Autodesk Inventor part; units mm, degrees
(part 5 of 7)
  arc A1272 (-12.9119, 20.5084) -> (-12.9119, 24.5084) centre (-12.9119, 22.5084) ccw
  arc A1273 (-46.3463, 24.5084) -> (-46.3463, 20.5084) centre (-46.3463, 22.5084) ccw
  arc A1274 (-52.9119, 20.5084) -> (-52.9119, 24.5084) centre (-52.9119, 22.5084) ccw
  arc A1275 (-46.3463, 24.5084) -> (-46.3463, 20.5084) centre (-46.3463, 22.5084) ccw
  arc A1276 (-46.3463, 24.5084) -> (-46.3463, 20.5084) centre (-46.3463, 22.5084) ccw
  arc A1277 (-46.3463, 24.5084) -> (-46.3463, 20.5084) centre (-46.3463, 22.5084) ccw
  arc A1278 (-46.3463, 24.5084) -> (-46.3463, 20.5084) centre (-46.3463, 22.5084) ccw
  arc A1279 (-46.3463, 24.5084) -> (-46.3463, 20.5084) centre (-46.3463, 22.5084) ccw
  arc A1280 (-52.9119, 20.5084) -> (-52.9119, 24.5084) centre (-52.9119, 22.5084) ccw
  arc A1281 (-52.9119, 20.5084) -> (-52.9119, 24.5084) centre (-52.9119, 22.5084) ccw
  arc A1282 (-52.9119, 20.5084) -> (-52.9119, 24.5084) centre (-52.9119, 22.5084) ccw
  arc A1283 (-52.9119, 20.5084) -> (-52.9119, 24.5084) centre (-52.9119, 22.5084) ccw
  line L1132 (-42.4124, 31.4654) -> (-55.8468, 31.4654)
  line L1133 (-55.8468, 27.4654) -> (-42.4124, 27.4654)
  line L1134 (-55.8468, 27.4654) -> (-42.4124, 27.4654)
  line L1135 (-55.8468, 27.4654) -> (-42.4124, 27.4654)
  line L1136 (-55.8468, 27.4654) -> (-42.4124, 27.4654)
  line L1137 (-55.8468, 27.4654) -> (-42.4124, 27.4654)
  line L1138 (-42.4124, 31.4654) -> (-55.8468, 31.4654)
  line L1139 (-42.4124, 31.4654) -> (-55.8468, 31.4654)
  line L1140 (-42.4124, 31.4654) -> (-55.8468, 31.4654)
  line L1141 (-42.4124, 31.4654) -> (-55.8468, 31.4654)
  arc A1284 (-86.3463, 24.5084) -> (-86.3463, 20.5084) centre (-86.3463, 22.5084) ccw
  arc A1285 (-86.3463, 24.5084) -> (-86.3463, 20.5084) centre (-86.3463, 22.5084) ccw
  arc A1286 (-86.3463, 24.5084) -> (-86.3463, 20.5084) centre (-86.3463, 22.5084) ccw
  arc A1287 (-92.9119, 20.5084) -> (-92.9119, 24.5084) centre (-92.9119, 22.5084) ccw
  line L1142 (-82.4124, 31.4654) -> (-95.8468, 31.4654)
  line L1143 (-95.8468, 27.4654) -> (-82.4124, 27.4654)
  line L1144 (-86.3463, 20.5084) -> (-72.9119, 20.5084)
  line L1145 (-86.3463, 20.5084) -> (-72.9119, 20.5084)
  line L1146 (-86.3463, 20.5084) -> (-72.9119, 20.5084)
  line L1147 (-72.9119, 24.5084) -> (-86.3463, 24.5084)
  line L1148 (-72.9119, 24.5084) -> (-86.3463, 24.5084)
  line L1149 (-72.9119, 24.5084) -> (-86.3463, 24.5084)
  arc A1288 (-75.8468, 31.4654) -> (-75.8468, 27.4654) centre (-75.8468, 29.4654) ccw
  arc A1289 (-75.8468, 31.4654) -> (-75.8468, 27.4654) centre (-75.8468, 29.4654) ccw
  arc A1290 (-75.8468, 31.4654) -> (-75.8468, 27.4654) centre (-75.8468, 29.4654) ccw
  arc A1291 (-75.8468, 31.4654) -> (-75.8468, 27.4654) centre (-75.8468, 29.4654) ccw
  arc A1292 (-82.4124, 27.4654) -> (-82.4124, 31.4654) centre (-82.4124, 29.4654) ccw
  line L1150 (-66.3463, 20.5084) -> (-52.9119, 20.5084)
  line L1151 (-52.9119, 24.5084) -> (-66.3463, 24.5084)
  line L1152 (-52.9119, 24.5084) -> (-66.3463, 24.5084)
  line L1153 (-66.3463, 20.5084) -> (-52.9119, 20.5084)
  line L1154 (-52.9119, 24.5084) -> (-66.3463, 24.5084)
  line L1155 (-52.9119, 24.5084) -> (-66.3463, 24.5084)
  line L1156 (-52.9119, 24.5084) -> (-66.3463, 24.5084)
  line L1157 (-66.3463, 20.5084) -> (-52.9119, 20.5084)
  line L1158 (-66.3463, 20.5084) -> (-52.9119, 20.5084)
  line L1159 (-66.3463, 20.5084) -> (-52.9119, 20.5084)
  line L1160 (-46.3463, 20.5084) -> (-32.9119, 20.5084)
  line L1161 (-32.9119, 24.5084) -> (-46.3463, 24.5084)
  line L1162 (-32.9119, 24.5084) -> (-46.3463, 24.5084)
  line L1163 (-46.3463, 20.5084) -> (-32.9119, 20.5084)
  line L1164 (-32.9119, 24.5084) -> (-46.3463, 24.5084)
  line L1165 (-32.9119, 24.5084) -> (-46.3463, 24.5084)
  line L1166 (-32.9119, 24.5084) -> (-46.3463, 24.5084)
  line L1167 (-46.3463, 20.5084) -> (-32.9119, 20.5084)
  line L1168 (-46.3463, 20.5084) -> (-32.9119, 20.5084)
  line L1169 (-46.3463, 20.5084) -> (-32.9119, 20.5084)
  line L1170 (-46.3463, 20.5084) -> (-32.9119, 20.5084)
  line L1171 (-32.9119, 24.5084) -> (-46.3463, 24.5084)
  arc A1293 (-55.8468, 31.4654) -> (-55.8468, 27.4654) centre (-55.8468, 29.4654) ccw
  arc A1294 (-55.8468, 31.4654) -> (-55.8468, 27.4654) centre (-55.8468, 29.4654) ccw
  arc A1295 (-55.8468, 31.4654) -> (-55.8468, 27.4654) centre (-55.8468, 29.4654) ccw
  arc A1296 (-62.4124, 27.4654) -> (-62.4124, 31.4654) centre (-62.4124, 29.4654) ccw
  arc A1297 (-55.8468, 31.4654) -> (-55.8468, 27.4654) centre (-55.8468, 29.4654) ccw
  arc A1298 (-55.8468, 31.4654) -> (-55.8468, 27.4654) centre (-55.8468, 29.4654) ccw
  arc A1299 (-55.8468, 31.4654) -> (-55.8468, 27.4654) centre (-55.8468, 29.4654) ccw
  arc A1300 (-55.8468, 31.4654) -> (-55.8468, 27.4654) centre (-55.8468, 29.4654) ccw
  arc A1301 (-62.4124, 27.4654) -> (-62.4124, 31.4654) centre (-62.4124, 29.4654) ccw
  arc A1302 (-62.4124, 27.4654) -> (-62.4124, 31.4654) centre (-62.4124, 29.4654) ccw
  arc A1303 (-66.3463, 24.5084) -> (-66.3463, 20.5084) centre (-66.3463, 22.5084) ccw
  arc A1304 (-72.9119, 20.5084) -> (-72.9119, 24.5084) centre (-72.9119, 22.5084) ccw
  arc A1305 (-66.3463, 24.5084) -> (-66.3463, 20.5084) centre (-66.3463, 22.5084) ccw
  line L1172 (-62.4124, 31.4654) -> (-75.8468, 31.4654)
  line L1173 (-75.8468, 27.4654) -> (-62.4124, 27.4654)
  arc A1306 (-72.9119, 20.5084) -> (-72.9119, 24.5084) centre (-72.9119, 22.5084) ccw
  line L1174 (-62.4124, 31.4654) -> (-75.8468, 31.4654)
  line L1175 (-75.8468, 27.4654) -> (-62.4124, 27.4654)
  arc A1307 (-66.3463, 24.5084) -> (-66.3463, 20.5084) centre (-66.3463, 22.5084) ccw
  arc A1308 (-66.3463, 24.5084) -> (-66.3463, 20.5084) centre (-66.3463, 22.5084) ccw
  arc A1309 (-66.3463, 24.5084) -> (-66.3463, 20.5084) centre (-66.3463, 22.5084) ccw
  line L1176 (-62.4124, 31.4654) -> (-75.8468, 31.4654)
  line L1177 (-75.8468, 27.4654) -> (-62.4124, 27.4654)
  arc A1310 (-72.9119, 20.5084) -> (-72.9119, 24.5084) centre (-72.9119, 22.5084) ccw
  arc A1311 (-106.3463, 24.5084) -> (-106.3463, 20.5084) centre (-106.3463, 22.5084) ccw
  arc A1312 (-95.8468, 31.4654) -> (-95.8468, 27.4654) centre (-95.8468, 29.4654) ccw
  line L1178 (-92.9119, 24.5084) -> (-106.3463, 24.5084)
  line L1179 (-106.3463, 20.5084) -> (-92.9119, 20.5084)
  arc A1313 (-35.8468, 31.4654) -> (-35.8468, 27.4654) centre (-35.8468, 29.4654) ccw
  arc A1314 (-35.8468, 31.4654) -> (-35.8468, 27.4654) centre (-35.8468, 29.4654) ccw
  arc A1315 (-35.8468, 31.4654) -> (-35.8468, 27.4654) centre (-35.8468, 29.4654) ccw
  arc A1316 (-42.4124, 27.4654) -> (-42.4124, 31.4654) centre (-42.4124, 29.4654) ccw
  arc A1317 (-42.4124, 27.4654) -> (-42.4124, 31.4654) centre (-42.4124, 29.4654) ccw
  arc A1318 (-35.8468, 31.4654) -> (-35.8468, 27.4654) centre (-35.8468, 29.4654) ccw
  arc A1319 (-35.8468, 31.4654) -> (-35.8468, 27.4654) centre (-35.8468, 29.4654) ccw
  arc A1320 (-35.8468, 31.4654) -> (-35.8468, 27.4654) centre (-35.8468, 29.4654) ccw
  arc A1321 (-35.8468, 31.4654) -> (-35.8468, 27.4654) centre (-35.8468, 29.4654) ccw
  arc A1322 (-35.8468, 31.4654) -> (-35.8468, 27.4654) centre (-35.8468, 29.4654) ccw
  arc A1323 (-35.8468, 31.4654) -> (-35.8468, 27.4654) centre (-35.8468, 29.4654) ccw
  arc A1324 (-42.4124, 27.4654) -> (-42.4124, 31.4654) centre (-42.4124, 29.4654) ccw
  arc A1325 (-42.4124, 27.4654) -> (-42.4124, 31.4654) centre (-42.4124, 29.4654) ccw
  arc A1326 (-42.4124, 27.4654) -> (-42.4124, 31.4654) centre (-42.4124, 29.4654) ccw
  arc A1327 (44.1532, 45.4654) -> (44.1532, 41.4654) centre (44.1532, 43.4654) ccw
  arc A1328 (44.1532, 45.4654) -> (44.1532, 41.4654) centre (44.1532, 43.4654) ccw
  arc A1329 (44.1532, 45.4654) -> (44.1532, 41.4654) centre (44.1532, 43.4654) ccw
  arc A1330 (44.1532, 45.4654) -> (44.1532, 41.4654) centre (44.1532, 43.4654) ccw
  arc A1331 (44.1532, 45.4654) -> (44.1532, 41.4654) centre (44.1532, 43.4654) ccw
  arc A1332 (44.1532, 45.4654) -> (44.1532, 41.4654) centre (44.1532, 43.4654) ccw
  arc A1333 (44.1532, 45.4654) -> (44.1532, 41.4654) centre (44.1532, 43.4654) ccw
  arc A1334 (33.6537, 38.5084) -> (33.6537, 34.5084) centre (33.6537, 36.5084) ccw
  arc A1335 (27.0881, 34.5084) -> (27.0881, 38.5084) centre (27.0881, 36.5084) ccw
  arc A1336 (27.0881, 34.5084) -> (27.0881, 38.5084) centre (27.0881, 36.5084) ccw
  arc A1337 (33.6537, 38.5084) -> (33.6537, 34.5084) centre (33.6537, 36.5084) ccw
  arc A1338 (27.0881, 34.5084) -> (27.0881, 38.5084) centre (27.0881, 36.5084) ccw
  arc A1339 (27.0881, 34.5084) -> (27.0881, 38.5084) centre (27.0881, 36.5084) ccw
  arc A1340 (27.0881, 34.5084) -> (27.0881, 38.5084) centre (27.0881, 36.5084) ccw
  arc A1341 (27.0881, 34.5084) -> (27.0881, 38.5084) centre (27.0881, 36.5084) ccw
  arc A1342 (33.6537, 38.5084) -> (33.6537, 34.5084) centre (33.6537, 36.5084) ccw
  arc A1343 (33.6537, 38.5084) -> (33.6537, 34.5084) centre (33.6537, 36.5084) ccw
  arc A1344 (33.6537, 38.5084) -> (33.6537, 34.5084) centre (33.6537, 36.5084) ccw
  line L1180 (24.1532, 41.4654) -> (37.5876, 41.4654)
  line L1181 (37.5876, 45.4654) -> (24.1532, 45.4654)
  line L1182 (24.1532, 41.4654) -> (37.5876, 41.4654)
  line L1183 (24.1532, 41.4654) -> (37.5876, 41.4654)
  line L1184 (24.1532, 41.4654) -> (37.5876, 41.4654)
  line L1185 (24.1532, 41.4654) -> (37.5876, 41.4654)
  line L1186 (24.1532, 41.4654) -> (37.5876, 41.4654)
  line L1187 (37.5876, 45.4654) -> (24.1532, 45.4654)
  line L1188 (37.5876, 45.4654) -> (24.1532, 45.4654)
  line L1189 (37.5876, 45.4654) -> (24.1532, 45.4654)
  line L1190 (37.5876, 45.4654) -> (24.1532, 45.4654)
  line L1191 (37.5876, 45.4654) -> (24.1532, 45.4654)
  arc A1345 (37.5876, 41.4654) -> (37.5876, 45.4654) centre (37.5876, 43.4654) ccw
  arc A1346 (37.5876, 41.4654) -> (37.5876, 45.4654) centre (37.5876, 43.4654) ccw
  arc A1347 (37.5876, 41.4654) -> (37.5876, 45.4654) centre (37.5876, 43.4654) ccw
  arc A1348 (37.5876, 41.4654) -> (37.5876, 45.4654) centre (37.5876, 43.4654) ccw
  arc A1349 (37.5876, 41.4654) -> (37.5876, 45.4654) centre (37.5876, 43.4654) ccw
  arc A1350 (37.5876, 41.4654) -> (37.5876, 45.4654) centre (37.5876, 43.4654) ccw
  arc A1351 (44.1532, 45.4654) -> (44.1532, 41.4654) centre (44.1532, 43.4654) ccw
  arc A1352 (47.0881, 34.5084) -> (47.0881, 38.5084) centre (47.0881, 36.5084) ccw
  arc A1353 (47.0881, 34.5084) -> (47.0881, 38.5084) centre (47.0881, 36.5084) ccw
  arc A1354 (53.6537, 38.5084) -> (53.6537, 34.5084) centre (53.6537, 36.5084) ccw
  arc A1355 (47.0881, 34.5084) -> (47.0881, 38.5084) centre (47.0881, 36.5084) ccw
  arc A1356 (47.0881, 34.5084) -> (47.0881, 38.5084) centre (47.0881, 36.5084) ccw
  arc A1357 (47.0881, 34.5084) -> (47.0881, 38.5084) centre (47.0881, 36.5084) ccw
  arc A1358 (53.6537, 38.5084) -> (53.6537, 34.5084) centre (53.6537, 36.5084) ccw
  arc A1359 (53.6537, 38.5084) -> (53.6537, 34.5084) centre (53.6537, 36.5084) ccw
  line L1192 (57.5876, 45.4654) -> (44.1532, 45.4654)
  line L1193 (44.1532, 41.4654) -> (57.5876, 41.4654)
  line L1194 (57.5876, 45.4654) -> (44.1532, 45.4654)
  line L1195 (44.1532, 41.4654) -> (57.5876, 41.4654)
  line L1196 (44.1532, 41.4654) -> (57.5876, 41.4654)
  line L1197 (44.1532, 41.4654) -> (57.5876, 41.4654)
  line L1198 (44.1532, 41.4654) -> (57.5876, 41.4654)
  line L1199 (57.5876, 45.4654) -> (44.1532, 45.4654)
  line L1200 (57.5876, 45.4654) -> (44.1532, 45.4654)
  line L1201 (57.5876, 45.4654) -> (44.1532, 45.4654)
  arc A1360 (57.5876, 41.4654) -> (57.5876, 45.4654) centre (57.5876, 43.4654) ccw
  arc A1361 (64.1532, 45.4654) -> (64.1532, 41.4654) centre (64.1532, 43.4654) ccw
  line L1202 (53.6537, 34.5084) -> (67.0881, 34.5084)
  line L1203 (53.6537, 34.5084) -> (67.0881, 34.5084)
  line L1204 (53.6537, 34.5084) -> (67.0881, 34.5084)
  line L1205 (67.0881, 38.5084) -> (53.6537, 38.5084)
  line L1206 (67.0881, 38.5084) -> (53.6537, 38.5084)
  line L1207 (67.0881, 38.5084) -> (53.6537, 38.5084)
  arc A1362 (64.1532, 45.4654) -> (64.1532, 41.4654) centre (64.1532, 43.4654) ccw
  arc A1363 (64.1532, 45.4654) -> (64.1532, 41.4654) centre (64.1532, 43.4654) ccw
  arc A1364 (64.1532, 45.4654) -> (64.1532, 41.4654) centre (64.1532, 43.4654) ccw
  arc A1365 (64.1532, 45.4654) -> (64.1532, 41.4654) centre (64.1532, 43.4654) ccw
  arc A1366 (57.5876, 41.4654) -> (57.5876, 45.4654) centre (57.5876, 43.4654) ccw
  arc A1367 (57.5876, 41.4654) -> (57.5876, 45.4654) centre (57.5876, 43.4654) ccw
  arc A1368 (57.5876, 41.4654) -> (57.5876, 45.4654) centre (57.5876, 43.4654) ccw
  arc A1369 (57.5876, 41.4654) -> (57.5876, 45.4654) centre (57.5876, 43.4654) ccw
  arc A1370 (67.0881, 34.5084) -> (67.0881, 38.5084) centre (67.0881, 36.5084) ccw
  arc A1371 (67.0881, 34.5084) -> (67.0881, 38.5084) centre (67.0881, 36.5084) ccw
  arc A1372 (67.0881, 34.5084) -> (67.0881, 38.5084) centre (67.0881, 36.5084) ccw
  line L1208 (77.5876, 45.4654) -> (64.1532, 45.4654)
  line L1209 (77.5876, 45.4654) -> (64.1532, 45.4654)
  line L1210 (77.5876, 45.4654) -> (64.1532, 45.4654)
  line L1211 (64.1532, 41.4654) -> (77.5876, 41.4654)
  line L1212 (64.1532, 41.4654) -> (77.5876, 41.4654)
  line L1213 (64.1532, 41.4654) -> (77.5876, 41.4654)
  arc A1373 (73.6537, 38.5084) -> (73.6537, 34.5084) centre (73.6537, 36.5084) ccw
  arc A1374 (77.5876, 41.4654) -> (77.5876, 45.4654) centre (77.5876, 43.4654) ccw
  arc A1375 (77.5876, 41.4654) -> (77.5876, 45.4654) centre (77.5876, 43.4654) ccw
  arc A1376 (77.5876, 41.4654) -> (77.5876, 45.4654) centre (77.5876, 43.4654) ccw
  arc A1377 (84.1532, 45.4654) -> (84.1532, 41.4654) centre (84.1532, 43.4654) ccw
  arc A1378 (84.1532, 45.4654) -> (84.1532, 41.4654) centre (84.1532, 43.4654) ccw
  line L1214 (87.0881, 38.5084) -> (73.6537, 38.5084)
  arc A1379 (87.0881, 34.5084) -> (87.0881, 38.5084) centre (87.0881, 36.5084) ccw
  line L1215 (73.6537, 34.5084) -> (87.0881, 34.5084)
  line L1216 (84.1532, 41.4654) -> (97.5876, 41.4654)
  line L1217 (97.5876, 45.4654) -> (84.1532, 45.4654)
  arc A1380 (97.5876, 41.4654) -> (97.5876, 45.4654) centre (97.5876, 43.4654) ccw
  line L1218 (33.6537, 34.5084) -> (47.0881, 34.5084)
  line L1219 (47.0881, 38.5084) -> (33.6537, 38.5084)
  line L1220 (33.6537, 34.5084) -> (47.0881, 34.5084)
  line L1221 (47.0881, 38.5084) -> (33.6537, 38.5084)
  line L1222 (47.0881, 38.5084) -> (33.6537, 38.5084)
  line L1223 (47.0881, 38.5084) -> (33.6537, 38.5084)
  line L1224 (47.0881, 38.5084) -> (33.6537, 38.5084)
  line L1225 (33.6537, 34.5084) -> (47.0881, 34.5084)
  line L1226 (33.6537, 34.5084) -> (47.0881, 34.5084)
  line L1227 (33.6537, 34.5084) -> (47.0881, 34.5084)
  arc A1381 (13.6537, 38.5084) -> (13.6537, 34.5084) centre (13.6537, 36.5084) ccw
  arc A1382 (13.6537, 38.5084) -> (13.6537, 34.5084) centre (13.6537, 36.5084) ccw
  arc A1383 (13.6537, 38.5084) -> (13.6537, 34.5084) centre (13.6537, 36.5084) ccw
  arc A1384 (13.6537, 38.5084) -> (13.6537, 34.5084) centre (13.6537, 36.5084) ccw
  arc A1385 (13.6537, 38.5084) -> (13.6537, 34.5084) centre (13.6537, 36.5084) ccw
  arc A1386 (13.6537, 38.5084) -> (13.6537, 34.5084) centre (13.6537, 36.5084) ccw
  arc A1387 (7.0881, 34.5084) -> (7.0881, 38.5084) centre (7.0881, 36.5084) ccw
  arc A1388 (7.0881, 34.5084) -> (7.0881, 38.5084) centre (7.0881, 36.5084) ccw
  arc A1389 (7.0881, 34.5084) -> (7.0881, 38.5084) centre (7.0881, 36.5084) ccw
  arc A1390 (7.0881, 34.5084) -> (7.0881, 38.5084) centre (7.0881, 36.5084) ccw
  arc A1391 (17.5876, 41.4654) -> (17.5876, 45.4654) centre (17.5876, 43.4654) ccw
  arc A1392 (17.5876, 41.4654) -> (17.5876, 45.4654) centre (17.5876, 43.4654) ccw
  arc A1393 (17.5876, 41.4654) -> (17.5876, 45.4654) centre (17.5876, 43.4654) ccw
  arc A1394 (17.5876, 41.4654) -> (17.5876, 45.4654) centre (17.5876, 43.4654) ccw
  arc A1395 (17.5876, 41.4654) -> (17.5876, 45.4654) centre (17.5876, 43.4654) ccw
  arc A1396 (17.5876, 41.4654) -> (17.5876, 45.4654) centre (17.5876, 43.4654) ccw
  arc A1397 (24.1532, 45.4654) -> (24.1532, 41.4654) centre (24.1532, 43.4654) ccw
  arc A1398 (24.1532, 45.4654) -> (24.1532, 41.4654) centre (24.1532, 43.4654) ccw
  arc A1399 (24.1532, 45.4654) -> (24.1532, 41.4654) centre (24.1532, 43.4654) ccw
  arc A1400 (24.1532, 45.4654) -> (24.1532, 41.4654) centre (24.1532, 43.4654) ccw
  arc A1401 (24.1532, 45.4654) -> (24.1532, 41.4654) centre (24.1532, 43.4654) ccw
  arc A1402 (24.1532, 45.4654) -> (24.1532, 41.4654) centre (24.1532, 43.4654) ccw
  arc A1403 (24.1532, 45.4654) -> (24.1532, 41.4654) centre (24.1532, 43.4654) ccw
  arc A1404 (24.1532, 45.4654) -> (24.1532, 41.4654) centre (24.1532, 43.4654) ccw
  arc A1405 (24.1532, 45.4654) -> (24.1532, 41.4654) centre (24.1532, 43.4654) ccw
  arc A1406 (4.1532, 45.4654) -> (4.1532, 41.4654) centre (4.1532, 43.4654) ccw
  arc A1407 (4.1532, 45.4654) -> (4.1532, 41.4654) centre (4.1532, 43.4654) ccw
  arc A1408 (4.1532, 45.4654) -> (4.1532, 41.4654) centre (4.1532, 43.4654) ccw
  arc A1409 (4.1532, 45.4654) -> (4.1532, 41.4654) centre (4.1532, 43.4654) ccw
  arc A1410 (4.1532, 45.4654) -> (4.1532, 41.4654) centre (4.1532, 43.4654) ccw
  arc A1411 (4.1532, 45.4654) -> (4.1532, 41.4654) centre (4.1532, 43.4654) ccw
  arc A1412 (4.1532, 45.4654) -> (4.1532, 41.4654) centre (4.1532, 43.4654) ccw
  arc A1413 (4.1532, 45.4654) -> (4.1532, 41.4654) centre (4.1532, 43.4654) ccw
  arc A1414 (4.1532, 45.4654) -> (4.1532, 41.4654) centre (4.1532, 43.4654) ccw
  arc A1415 (-2.4124, 41.4654) -> (-2.4124, 45.4654) centre (-2.4124, 43.4654) ccw
  arc A1416 (-2.4124, 41.4654) -> (-2.4124, 45.4654) centre (-2.4124, 43.4654) ccw
  arc A1417 (-2.4124, 41.4654) -> (-2.4124, 45.4654) centre (-2.4124, 43.4654) ccw
  arc A1418 (-2.4124, 41.4654) -> (-2.4124, 45.4654) centre (-2.4124, 43.4654) ccw
  arc A1419 (-32.9119, 34.5084) -> (-32.9119, 38.5084) centre (-32.9119, 36.5084) ccw
  arc A1420 (-32.9119, 34.5084) -> (-32.9119, 38.5084) centre (-32.9119, 36.5084) ccw
  arc A1421 (-32.9119, 34.5084) -> (-32.9119, 38.5084) centre (-32.9119, 36.5084) ccw
  arc A1422 (-32.9119, 34.5084) -> (-32.9119, 38.5084) centre (-32.9119, 36.5084) ccw
  arc A1423 (-32.9119, 34.5084) -> (-32.9119, 38.5084) centre (-32.9119, 36.5084) ccw
  arc A1424 (-32.9119, 34.5084) -> (-32.9119, 38.5084) centre (-32.9119, 36.5084) ccw
  line L1228 (27.0881, 38.5084) -> (13.6537, 38.5084)
  line L1229 (13.6537, 34.5084) -> (27.0881, 34.5084)
  line L1230 (27.0881, 38.5084) -> (13.6537, 38.5084)
  line L1231 (13.6537, 34.5084) -> (27.0881, 34.5084)
  line L1232 (13.6537, 34.5084) -> (27.0881, 34.5084)
  line L1233 (27.0881, 38.5084) -> (13.6537, 38.5084)
  line L1234 (27.0881, 38.5084) -> (13.6537, 38.5084)
  line L1235 (27.0881, 38.5084) -> (13.6537, 38.5084)
  line L1236 (13.6537, 34.5084) -> (27.0881, 34.5084)
  line L1237 (13.6537, 34.5084) -> (27.0881, 34.5084)
  line L1238 (13.6537, 34.5084) -> (27.0881, 34.5084)
  line L1239 (27.0881, 38.5084) -> (13.6537, 38.5084)
  line L1240 (4.1532, 41.4654) -> (17.5876, 41.4654)
  line L1241 (4.1532, 41.4654) -> (17.5876, 41.4654)
  line L1242 (4.1532, 41.4654) -> (17.5876, 41.4654)
  line L1243 (4.1532, 41.4654) -> (17.5876, 41.4654)
  line L1244 (4.1532, 41.4654) -> (17.5876, 41.4654)
  line L1245 (4.1532, 41.4654) -> (17.5876, 41.4654)
  line L1246 (17.5876, 45.4654) -> (4.1532, 45.4654)
  line L1247 (17.5876, 45.4654) -> (4.1532, 45.4654)
  line L1248 (17.5876, 45.4654) -> (4.1532, 45.4654)
  line L1249 (17.5876, 45.4654) -> (4.1532, 45.4654)
  line L1250 (17.5876, 45.4654) -> (4.1532, 45.4654)
  line L1251 (17.5876, 45.4654) -> (4.1532, 45.4654)
  arc A1425 (7.0881, 34.5084) -> (7.0881, 38.5084) centre (7.0881, 36.5084) ccw
  arc A1426 (7.0881, 34.5084) -> (7.0881, 38.5084) centre (7.0881, 36.5084) ccw
  line L1252 (-6.3463, 34.5084) -> (7.0881, 34.5084)
  line L1253 (7.0881, 38.5084) -> (-6.3463, 38.5084)
  line L1254 (7.0881, 38.5084) -> (-6.3463, 38.5084)
  line L1255 (-6.3463, 34.5084) -> (7.0881, 34.5084)
  line L1256 (-6.3463, 34.5084) -> (7.0881, 34.5084)
  line L1257 (7.0881, 38.5084) -> (-6.3463, 38.5084)
  line L1258 (7.0881, 38.5084) -> (-6.3463, 38.5084)
  line L1259 (7.0881, 38.5084) -> (-6.3463, 38.5084)
  line L1260 (-6.3463, 34.5084) -> (7.0881, 34.5084)
  line L1261 (-6.3463, 34.5084) -> (7.0881, 34.5084)
  line L1262 (-6.3463, 34.5084) -> (7.0881, 34.5084)
  line L1263 (7.0881, 38.5084) -> (-6.3463, 38.5084)
  arc A1427 (-6.3463, 38.5084) -> (-6.3463, 34.5084) centre (-6.3463, 36.5084) ccw
  arc A1428 (-6.3463, 38.5084) -> (-6.3463, 34.5084) centre (-6.3463, 36.5084) ccw
  arc A1429 (-6.3463, 38.5084) -> (-6.3463, 34.5084) centre (-6.3463, 36.5084) ccw
  arc A1430 (-6.3463, 38.5084) -> (-6.3463, 34.5084) centre (-6.3463, 36.5084) ccw
  arc A1431 (-6.3463, 38.5084) -> (-6.3463, 34.5084) centre (-6.3463, 36.5084) ccw
  arc A1432 (-6.3463, 38.5084) -> (-6.3463, 34.5084) centre (-6.3463, 36.5084) ccw
  arc A1433 (-12.9119, 34.5084) -> (-12.9119, 38.5084) centre (-12.9119, 36.5084) ccw
  arc A1434 (-12.9119, 34.5084) -> (-12.9119, 38.5084) centre (-12.9119, 36.5084) ccw
  arc A1435 (-12.9119, 34.5084) -> (-12.9119, 38.5084) centre (-12.9119, 36.5084) ccw
  arc A1436 (-12.9119, 34.5084) -> (-12.9119, 38.5084) centre (-12.9119, 36.5084) ccw
  arc A1437 (-12.9119, 34.5084) -> (-12.9119, 38.5084) centre (-12.9119, 36.5084) ccw
  line L1264 (-2.4124, 45.4654) -> (-15.8468, 45.4654)
  line L1265 (-15.8468, 41.4654) -> (-2.4124, 41.4654)
  line L1266 (-2.4124, 45.4654) -> (-15.8468, 45.4654)
  line L1267 (-15.8468, 41.4654) -> (-2.4124, 41.4654)
  line L1268 (-2.4124, 45.4654) -> (-15.8468, 45.4654)
  line L1269 (-15.8468, 41.4654) -> (-2.4124, 41.4654)
  line L1270 (-2.4124, 45.4654) -> (-15.8468, 45.4654)
  line L1271 (-15.8468, 41.4654) -> (-2.4124, 41.4654)
  line L1272 (-2.4124, 45.4654) -> (-15.8468, 45.4654)
  line L1273 (-15.8468, 41.4654) -> (-2.4124, 41.4654)
  line L1274 (-15.8468, 41.4654) -> (-2.4124, 41.4654)
  line L1275 (-2.4124, 45.4654) -> (-15.8468, 45.4654)
  arc A1438 (-2.4124, 41.4654) -> (-2.4124, 45.4654) centre (-2.4124, 43.4654) ccw
  arc A1439 (-2.4124, 41.4654) -> (-2.4124, 45.4654) centre (-2.4124, 43.4654) ccw
  arc A1440 (-15.8468, 45.4654) -> (-15.8468, 41.4654) centre (-15.8468, 43.4654) ccw
  arc A1441 (-15.8468, 45.4654) -> (-15.8468, 41.4654) centre (-15.8468, 43.4654) ccw
  arc A1442 (-15.8468, 45.4654) -> (-15.8468, 41.4654) centre (-15.8468, 43.4654) ccw
  arc A1443 (-15.8468, 45.4654) -> (-15.8468, 41.4654) centre (-15.8468, 43.4654) ccw
  arc A1444 (-15.8468, 45.4654) -> (-15.8468, 41.4654) centre (-15.8468, 43.4654) ccw
  arc A1445 (-22.4124, 41.4654) -> (-22.4124, 45.4654) centre (-22.4124, 43.4654) ccw
  arc A1446 (-22.4124, 41.4654) -> (-22.4124, 45.4654) centre (-22.4124, 43.4654) ccw
  arc A1447 (-15.8468, 45.4654) -> (-15.8468, 41.4654) centre (-15.8468, 43.4654) ccw
  arc A1448 (-15.8468, 45.4654) -> (-15.8468, 41.4654) centre (-15.8468, 43.4654) ccw
  arc A1449 (-22.4124, 41.4654) -> (-22.4124, 45.4654) centre (-22.4124, 43.4654) ccw
  arc A1450 (-15.8468, 45.4654) -> (-15.8468, 41.4654) centre (-15.8468, 43.4654) ccw
  arc A1451 (-15.8468, 45.4654) -> (-15.8468, 41.4654) centre (-15.8468, 43.4654) ccw
  arc A1452 (-22.4124, 41.4654) -> (-22.4124, 45.4654) centre (-22.4124, 43.4654) ccw
  arc A1453 (-22.4124, 41.4654) -> (-22.4124, 45.4654) centre (-22.4124, 43.4654) ccw
  arc A1454 (-22.4124, 41.4654) -> (-22.4124, 45.4654) centre (-22.4124, 43.4654) ccw
  arc A1455 (-26.3463, 38.5084) -> (-26.3463, 34.5084) centre (-26.3463, 36.5084) ccw
  arc A1456 (-26.3463, 38.5084) -> (-26.3463, 34.5084) centre (-26.3463, 36.5084) ccw
  arc A1457 (-26.3463, 38.5084) -> (-26.3463, 34.5084) centre (-26.3463, 36.5084) ccw
  arc A1458 (-26.3463, 38.5084) -> (-26.3463, 34.5084) centre (-26.3463, 36.5084) ccw
  arc A1459 (-26.3463, 38.5084) -> (-26.3463, 34.5084) centre (-26.3463, 36.5084) ccw
  arc A1460 (-26.3463, 38.5084) -> (-26.3463, 34.5084) centre (-26.3463, 36.5084) ccw
  line L1276 (-35.8468, 41.4654) -> (-22.4124, 41.4654)
  line L1277 (-35.8468, 41.4654) -> (-22.4124, 41.4654)
  line L1278 (-35.8468, 41.4654) -> (-22.4124, 41.4654)
  line L1279 (-35.8468, 41.4654) -> (-22.4124, 41.4654)
  line L1280 (-35.8468, 41.4654) -> (-22.4124, 41.4654)
  line L1281 (-35.8468, 41.4654) -> (-22.4124, 41.4654)
  line L1282 (-22.4124, 45.4654) -> (-35.8468, 45.4654)
  line L1283 (-22.4124, 45.4654) -> (-35.8468, 45.4654)
  line L1284 (-22.4124, 45.4654) -> (-35.8468, 45.4654)
  line L1285 (-22.4124, 45.4654) -> (-35.8468, 45.4654)
  line L1286 (-22.4124, 45.4654) -> (-35.8468, 45.4654)
  line L1287 (-22.4124, 45.4654) -> (-35.8468, 45.4654)
  line L1288 (-26.3463, 34.5084) -> (-12.9119, 34.5084)
  line L1289 (-12.9119, 38.5084) -> (-26.3463, 38.5084)
  line L1290 (-12.9119, 38.5084) -> (-26.3463, 38.5084)
  line L1291 (-26.3463, 34.5084) -> (-12.9119, 34.5084)
  line L1292 (-12.9119, 38.5084) -> (-26.3463, 38.5084)
  line L1293 (-12.9119, 38.5084) -> (-26.3463, 38.5084)
  line L1294 (-26.3463, 34.5084) -> (-12.9119, 34.5084)
  line L1295 (-12.9119, 38.5084) -> (-26.3463, 38.5084)
  line L1296 (-12.9119, 38.5084) -> (-26.3463, 38.5084)
  line L1297 (-26.3463, 34.5084) -> (-12.9119, 34.5084)
  line L1298 (-26.3463, 34.5084) -> (-12.9119, 34.5084)
  line L1299 (-26.3463, 34.5084) -> (-12.9119, 34.5084)
  arc A1461 (-12.9119, 34.5084) -> (-12.9119, 38.5084) centre (-12.9119, 36.5084) ccw
  arc A1462 (-46.3463, 38.5084) -> (-46.3463, 34.5084) centre (-46.3463, 36.5084) ccw
  arc A1463 (-52.9119, 34.5084) -> (-52.9119, 38.5084) centre (-52.9119, 36.5084) ccw
  arc A1464 (-46.3463, 38.5084) -> (-46.3463, 34.5084) centre (-46.3463, 36.5084) ccw
  arc A1465 (-46.3463, 38.5084) -> (-46.3463, 34.5084) centre (-46.3463, 36.5084) ccw
  arc A1466 (-46.3463, 38.5084) -> (-46.3463, 34.5084) centre (-46.3463, 36.5084) ccw
  arc A1467 (-46.3463, 38.5084) -> (-46.3463, 34.5084) centre (-46.3463, 36.5084) ccw
  arc A1468 (-46.3463, 38.5084) -> (-46.3463, 34.5084) centre (-46.3463, 36.5084) ccw
  arc A1469 (-52.9119, 34.5084) -> (-52.9119, 38.5084) centre (-52.9119, 36.5084) ccw
  arc A1470 (-52.9119, 34.5084) -> (-52.9119, 38.5084) centre (-52.9119, 36.5084) ccw
  arc A1471 (-52.9119, 34.5084) -> (-52.9119, 38.5084) centre (-52.9119, 36.5084) ccw
  arc A1472 (-52.9119, 34.5084) -> (-52.9119, 38.5084) centre (-52.9119, 36.5084) ccw
  line L1300 (-42.4124, 45.4654) -> (-55.8468, 45.4654)
  line L1301 (-55.8468, 41.4654) -> (-42.4124, 41.4654)
  line L1302 (-55.8468, 41.4654) -> (-42.4124, 41.4654)
  line L1303 (-55.8468, 41.4654) -> (-42.4124, 41.4654)
  line L1304 (-55.8468, 41.4654) -> (-42.4124, 41.4654)
  line L1305 (-55.8468, 41.4654) -> (-42.4124, 41.4654)
  line L1306 (-42.4124, 45.4654) -> (-55.8468, 45.4654)
  line L1307 (-42.4124, 45.4654) -> (-55.8468, 45.4654)
  line L1308 (-42.4124, 45.4654) -> (-55.8468, 45.4654)
  line L1309 (-42.4124, 45.4654) -> (-55.8468, 45.4654)
  arc A1473 (-86.3463, 38.5084) -> (-86.3463, 34.5084) centre (-86.3463, 36.5084) ccw
  arc A1474 (-86.3463, 38.5084) -> (-86.3463, 34.5084) centre (-86.3463, 36.5084) ccw
  arc A1475 (-86.3463, 38.5084) -> (-86.3463, 34.5084) centre (-86.3463, 36.5084) ccw
  arc A1476 (-92.9119, 34.5084) -> (-92.9119, 38.5084) centre (-92.9119, 36.5084) ccw
  line L1310 (-82.4124, 45.4654) -> (-95.8468, 45.4654)
  line L1311 (-95.8468, 41.4654) -> (-82.4124, 41.4654)
  line L1312 (-86.3463, 34.5084) -> (-72.9119, 34.5084)
  line L1313 (-86.3463, 34.5084) -> (-72.9119, 34.5084)
  line L1314 (-86.3463, 34.5084) -> (-72.9119, 34.5084)
  line L1315 (-72.9119, 38.5084) -> (-86.3463, 38.5084)
  line L1316 (-72.9119, 38.5084) -> (-86.3463, 38.5084)
  line L1317 (-72.9119, 38.5084) -> (-86.3463, 38.5084)
  arc A1477 (-75.8468, 45.4654) -> (-75.8468, 41.4654) centre (-75.8468, 43.4654) ccw
  arc A1478 (-75.8468, 45.4654) -> (-75.8468, 41.4654) centre (-75.8468, 43.4654) ccw
  arc A1479 (-75.8468, 45.4654) -> (-75.8468, 41.4654) centre (-75.8468, 43.4654) ccw
  arc A1480 (-75.8468, 45.4654) -> (-75.8468, 41.4654) centre (-75.8468, 43.4654) ccw
  arc A1481 (-82.4124, 41.4654) -> (-82.4124, 45.4654) centre (-82.4124, 43.4654) ccw
  line L1318 (-66.3463, 34.5084) -> (-52.9119, 34.5084)
  line L1319 (-52.9119, 38.5084) -> (-66.3463, 38.5084)
  line L1320 (-52.9119, 38.5084) -> (-66.3463, 38.5084)
  line L1321 (-66.3463, 34.5084) -> (-52.9119, 34.5084)
  line L1322 (-52.9119, 38.5084) -> (-66.3463, 38.5084)
  line L1323 (-52.9119, 38.5084) -> (-66.3463, 38.5084)
  line L1324 (-52.9119, 38.5084) -> (-66.3463, 38.5084)
  line L1325 (-66.3463, 34.5084) -> (-52.9119, 34.5084)
  line L1326 (-66.3463, 34.5084) -> (-52.9119, 34.5084)
  line L1327 (-66.3463, 34.5084) -> (-52.9119, 34.5084)
  line L1328 (-46.3463, 34.5084) -> (-32.9119, 34.5084)
  line L1329 (-32.9119, 38.5084) -> (-46.3463, 38.5084)
  line L1330 (-32.9119, 38.5084) -> (-46.3463, 38.5084)
  line L1331 (-46.3463, 34.5084) -> (-32.9119, 34.5084)
  line L1332 (-32.9119, 38.5084) -> (-46.3463, 38.5084)
  line L1333 (-32.9119, 38.5084) -> (-46.3463, 38.5084)
  line L1334 (-32.9119, 38.5084) -> (-46.3463, 38.5084)
  line L1335 (-46.3463, 34.5084) -> (-32.9119, 34.5084)
  line L1336 (-46.3463, 34.5084) -> (-32.9119, 34.5084)
  line L1337 (-46.3463, 34.5084) -> (-32.9119, 34.5084)
  line L1338 (-46.3463, 34.5084) -> (-32.9119, 34.5084)
  line L1339 (-32.9119, 38.5084) -> (-46.3463, 38.5084)
  arc A1482 (-55.8468, 45.4654) -> (-55.8468, 41.4654) centre (-55.8468, 43.4654) ccw
  arc A1483 (-55.8468, 45.4654) -> (-55.8468, 41.4654) centre (-55.8468, 43.4654) ccw
  arc A1484 (-55.8468, 45.4654) -> (-55.8468, 41.4654) centre (-55.8468, 43.4654) ccw
  arc A1485 (-62.4124, 41.4654) -> (-62.4124, 45.4654) centre (-62.4124, 43.4654) ccw
  arc A1486 (-55.8468, 45.4654) -> (-55.8468, 41.4654) centre (-55.8468, 43.4654) ccw
  arc A1487 (-55.8468, 45.4654) -> (-55.8468, 41.4654) centre (-55.8468, 43.4654) ccw
  arc A1488 (-55.8468, 45.4654) -> (-55.8468, 41.4654) centre (-55.8468, 43.4654) ccw
  arc A1489 (-55.8468, 45.4654) -> (-55.8468, 41.4654) centre (-55.8468, 43.4654) ccw
  arc A1490 (-62.4124, 41.4654) -> (-62.4124, 45.4654) centre (-62.4124, 43.4654) ccw
  arc A1491 (-62.4124, 41.4654) -> (-62.4124, 45.4654) centre (-62.4124, 43.4654) ccw
  arc A1492 (-66.3463, 38.5084) -> (-66.3463, 34.5084) centre (-66.3463, 36.5084) ccw
  arc A1493 (-72.9119, 34.5084) -> (-72.9119, 38.5084) centre (-72.9119, 36.5084) ccw
  arc A1494 (-66.3463, 38.5084) -> (-66.3463, 34.5084) centre (-66.3463, 36.5084) ccw
  line L1340 (-62.4124, 45.4654) -> (-75.8468, 45.4654)
  line L1341 (-75.8468, 41.4654) -> (-62.4124, 41.4654)
  arc A1495 (-72.9119, 34.5084) -> (-72.9119, 38.5084) centre (-72.9119, 36.5084) ccw
  line L1342 (-62.4124, 45.4654) -> (-75.8468, 45.4654)
  line L1343 (-75.8468, 41.4654) -> (-62.4124, 41.4654)
  arc A1496 (-66.3463, 38.5084) -> (-66.3463, 34.5084) centre (-66.3463, 36.5084) ccw
  arc A1497 (-66.3463, 38.5084) -> (-66.3463, 34.5084) centre (-66.3463, 36.5084) ccw
  arc A1498 (-66.3463, 38.5084) -> (-66.3463, 34.5084) centre (-66.3463, 36.5084) ccw
  line L1344 (-62.4124, 45.4654) -> (-75.8468, 45.4654)
  line L1345 (-75.8468, 41.4654) -> (-62.4124, 41.4654)
  arc A1499 (-72.9119, 34.5084) -> (-72.9119, 38.5084) centre (-72.9119, 36.5084) ccw
  arc A1500 (-106.3463, 38.5084) -> (-106.3463, 34.5084) centre (-106.3463, 36.5084) ccw
  arc A1501 (-95.8468, 45.4654) -> (-95.8468, 41.4654) centre (-95.8468, 43.4654) ccw
  line L1346 (-92.9119, 38.5084) -> (-106.3463, 38.5084)
  line L1347 (-106.3463, 34.5084) -> (-92.9119, 34.5084)
  arc A1502 (-35.8468, 45.4654) -> (-35.8468, 41.4654) centre (-35.8468, 43.4654) ccw
  arc A1503 (-35.8468, 45.4654) -> (-35.8468, 41.4654) centre (-35.8468, 43.4654) ccw
  arc A1504 (-35.8468, 45.4654) -> (-35.8468, 41.4654) centre (-35.8468, 43.4654) ccw
  arc A1505 (-42.4124, 41.4654) -> (-42.4124, 45.4654) centre (-42.4124, 43.4654) ccw
  arc A1506 (-42.4124, 41.4654) -> (-42.4124, 45.4654) centre (-42.4124, 43.4654) ccw
  arc A1507 (-35.8468, 45.4654) -> (-35.8468, 41.4654) centre (-35.8468, 43.4654) ccw
  arc A1508 (-35.8468, 45.4654) -> (-35.8468, 41.4654) centre (-35.8468, 43.4654) ccw
  arc A1509 (-35.8468, 45.4654) -> (-35.8468, 41.4654) centre (-35.8468, 43.4654) ccw
  arc A1510 (-35.8468, 45.4654) -> (-35.8468, 41.4654) centre (-35.8468, 43.4654) ccw
  arc A1511 (-35.8468, 45.4654) -> (-35.8468, 41.4654) centre (-35.8468, 43.4654) ccw
  arc A1512 (-35.8468, 45.4654) -> (-35.8468, 41.4654) centre (-35.8468, 43.4654) ccw
  arc A1513 (-42.4124, 41.4654) -> (-42.4124, 45.4654) centre (-42.4124, 43.4654) ccw
  arc A1514 (-42.4124, 41.4654) -> (-42.4124, 45.4654) centre (-42.4124, 43.4654) ccw
  arc A1515 (-42.4124, 41.4654) -> (-42.4124, 45.4654) centre (-42.4124, 43.4654) ccw
  arc A1516 (44.1532, 59.4654) -> (44.1532, 55.4654) centre (44.1532, 57.4654) ccw
  arc A1517 (44.1532, 59.4654) -> (44.1532, 55.4654) centre (44.1532, 57.4654) ccw
  arc A1518 (44.1532, 59.4654) -> (44.1532, 55.4654) centre (44.1532, 57.4654) ccw
  arc A1519 (44.1532, 59.4654) -> (44.1532, 55.4654) centre (44.1532, 57.4654) ccw
  arc A1520 (44.1532, 59.4654) -> (44.1532, 55.4654) centre (44.1532, 57.4654) ccw
  arc A1521 (44.1532, 59.4654) -> (44.1532, 55.4654) centre (44.1532, 57.4654) ccw
  arc A1522 (44.1532, 59.4654) -> (44.1532, 55.4654) centre (44.1532, 57.4654) ccw
  arc A1523 (33.6537, 52.5084) -> (33.6537, 48.5084) centre (33.6537, 50.5084) ccw
  arc A1524 (27.0881, 48.5084) -> (27.0881, 52.5084) centre (27.0881, 50.5084) ccw
  arc A1525 (27.0881, 48.5084) -> (27.0881, 52.5084) centre (27.0881, 50.5084) ccw
  arc A1526 (33.6537, 52.5084) -> (33.6537, 48.5084) centre (33.6537, 50.5084) ccw
  arc A1527 (27.0881, 48.5084) -> (27.0881, 52.5084) centre (27.0881, 50.5084) ccw
  arc A1528 (27.0881, 48.5084) -> (27.0881, 52.5084) centre (27.0881, 50.5084) ccw
  arc A1529 (27.0881, 48.5084) -> (27.0881, 52.5084) centre (27.0881, 50.5084) ccw
  arc A1530 (27.0881, 48.5084) -> (27.0881, 52.5084) centre (27.0881, 50.5084) ccw
  arc A1531 (33.6537, 52.5084) -> (33.6537, 48.5084) centre (33.6537, 50.5084) ccw
  arc A1532 (33.6537, 52.5084) -> (33.6537, 48.5084) centre (33.6537, 50.5084) ccw
  arc A1533 (33.6537, 52.5084) -> (33.6537, 48.5084) centre (33.6537, 50.5084) ccw
  line L1348 (24.1532, 55.4654) -> (37.5876, 55.4654)
  line L1349 (37.5876, 59.4654) -> (24.1532, 59.4654)
  line L1350 (24.1532, 55.4654) -> (37.5876, 55.4654)
  line L1351 (24.1532, 55.4654) -> (37.5876, 55.4654)
  line L1352 (24.1532, 55.4654) -> (37.5876, 55.4654)
  line L1353 (24.1532, 55.4654) -> (37.5876, 55.4654)
  line L1354 (24.1532, 55.4654) -> (37.5876, 55.4654)
  line L1355 (37.5876, 59.4654) -> (24.1532, 59.4654)
  line L1356 (37.5876, 59.4654) -> (24.1532, 59.4654)
  line L1357 (37.5876, 59.4654) -> (24.1532, 59.4654)
  line L1358 (37.5876, 59.4654) -> (24.1532, 59.4654)
  line L1359 (37.5876, 59.4654) -> (24.1532, 59.4654)
  arc A1534 (37.5876, 55.4654) -> (37.5876, 59.4654) centre (37.5876, 57.4654) ccw
  arc A1535 (37.5876, 55.4654) -> (37.5876, 59.4654) centre (37.5876, 57.4654) ccw
  arc A1536 (37.5876, 55.4654) -> (37.5876, 59.4654) centre (37.5876, 57.4654) ccw
  arc A1537 (37.5876, 55.4654) -> (37.5876, 59.4654) centre (37.5876, 57.4654) ccw
  arc A1538 (37.5876, 55.4654) -> (37.5876, 59.4654) centre (37.5876, 57.4654) ccw
  arc A1539 (37.5876, 55.4654) -> (37.5876, 59.4654) centre (37.5876, 57.4654) ccw
  arc A1540 (44.1532, 59.4654) -> (44.1532, 55.4654) centre (44.1532, 57.4654) ccw
  arc A1541 (47.0881, 48.5084) -> (47.0881, 52.5084) centre (47.0881, 50.5084) ccw
  arc A1542 (47.0881, 48.5084) -> (47.0881, 52.5084) centre (47.0881, 50.5084) ccw
  arc A1543 (53.6537, 52.5084) -> (53.6537, 48.5084) centre (53.6537, 50.5084) ccw
  arc A1544 (47.0881, 48.5084) -> (47.0881, 52.5084) centre (47.0881, 50.5084) ccw
  arc A1545 (47.0881, 48.5084) -> (47.0881, 52.5084) centre (47.0881, 50.5084) ccw
  arc A1546 (47.0881, 48.5084) -> (47.0881, 52.5084) centre (47.0881, 50.5084) ccw
  arc A1547 (53.6537, 52.5084) -> (53.6537, 48.5084) centre (53.6537, 50.5084) ccw
  arc A1548 (53.6537, 52.5084) -> (53.6537, 48.5084) centre (53.6537, 50.5084) ccw
  line L1360 (57.5876, 59.4654) -> (44.1532, 59.4654)
  line L1361 (44.1532, 55.4654) -> (57.5876, 55.4654)
  line L1362 (57.5876, 59.4654) -> (44.1532, 59.4654)
  line L1363 (44.1532, 55.4654) -> (57.5876, 55.4654)
  line L1364 (44.1532, 55.4654) -> (57.5876, 55.4654)
  line L1365 (44.1532, 55.4654) -> (57.5876, 55.4654)
  line L1366 (44.1532, 55.4654) -> (57.5876, 55.4654)
  line L1367 (57.5876, 59.4654) -> (44.1532, 59.4654)
  line L1368 (57.5876, 59.4654) -> (44.1532, 59.4654)
  line L1369 (57.5876, 59.4654) -> (44.1532, 59.4654)
  arc A1549 (57.5876, 55.4654) -> (57.5876, 59.4654) centre (57.5876, 57.4654) ccw
  arc A1550 (64.1532, 59.4654) -> (64.1532, 55.4654) centre (64.1532, 57.4654) ccw
  line L1370 (53.6537, 48.5084) -> (67.0881, 48.5084)
  line L1371 (53.6537, 48.5084) -> (67.0881, 48.5084)
  line L1372 (53.6537, 48.5084) -> (67.0881, 48.5084)
  line L1373 (67.0881, 52.5084) -> (53.6537, 52.5084)
  line L1374 (67.0881, 52.5084) -> (53.6537, 52.5084)
  line L1375 (67.0881, 52.5084) -> (53.6537, 52.5084)
  arc A1551 (64.1532, 59.4654) -> (64.1532, 55.4654) centre (64.1532, 57.4654) ccw
  arc A1552 (64.1532, 59.4654) -> (64.1532, 55.4654) centre (64.1532, 57.4654) ccw
  arc A1553 (64.1532, 59.4654) -> (64.1532, 55.4654) centre (64.1532, 57.4654) ccw
  arc A1554 (64.1532, 59.4654) -> (64.1532, 55.4654) centre (64.1532, 57.4654) ccw
  arc A1555 (57.5876, 55.4654) -> (57.5876, 59.4654) centre (57.5876, 57.4654) ccw
  arc A1556 (57.5876, 55.4654) -> (57.5876, 59.4654) centre (57.5876, 57.4654) ccw
  arc A1557 (57.5876, 55.4654) -> (57.5876, 59.4654) centre (57.5876, 57.4654) ccw
  arc A1558 (57.5876, 55.4654) -> (57.5876, 59.4654) centre (57.5876, 57.4654) ccw
  arc A1559 (67.0881, 48.5084) -> (67.0881, 52.5084) centre (67.0881, 50.5084) ccw
  arc A1560 (67.0881, 48.5084) -> (67.0881, 52.5084) centre (67.0881, 50.5084) ccw
  arc A1561 (67.0881, 48.5084) -> (67.0881, 52.5084) centre (67.0881, 50.5084) ccw
  line L1376 (77.5876, 59.4654) -> (64.1532, 59.4654)
  line L1377 (77.5876, 59.4654) -> (64.1532, 59.4654)
  line L1378 (77.5876, 59.4654) -> (64.1532, 59.4654)
  line L1379 (64.1532, 55.4654) -> (77.5876, 55.4654)
  line L1380 (64.1532, 55.4654) -> (77.5876, 55.4654)
  line L1381 (64.1532, 55.4654) -> (77.5876, 55.4654)
  arc A1562 (73.6537, 52.5084) -> (73.6537, 48.5084) centre (73.6537, 50.5084) ccw
  arc A1563 (77.5876, 55.4654) -> (77.5876, 59.4654) centre (77.5876, 57.4654) ccw
  arc A1564 (77.5876, 55.4654) -> (77.5876, 59.4654) centre (77.5876, 57.4654) ccw
  arc A1565 (77.5876, 55.4654) -> (77.5876, 59.4654) centre (77.5876, 57.4654) ccw
  arc A1566 (84.1532, 59.4654) -> (84.1532, 55.4654) centre (84.1532, 57.4654) ccw
  arc A1567 (84.1532, 59.4654) -> (84.1532, 55.4654) centre (84.1532, 57.4654) ccw
  line L1382 (87.0881, 52.5084) -> (73.6537, 52.5084)
  arc A1568 (87.0881, 48.5084) -> (87.0881, 52.5084) centre (87.0881, 50.5084) ccw
  line L1383 (73.6537, 48.5084) -> (87.0881, 48.5084)
  line L1384 (84.1532, 55.4654) -> (97.5876, 55.4654)
  line L1385 (97.5876, 59.4654) -> (84.1532, 59.4654)
  arc A1569 (97.5876, 55.4654) -> (97.5876, 59.4654) centre (97.5876, 57.4654) ccw
  line L1386 (33.6537, 48.5084) -> (47.0881, 48.5084)
  line L1387 (47.0881, 52.5084) -> (33.6537, 52.5084)
  line L1388 (33.6537, 48.5084) -> (47.0881, 48.5084)
  line L1389 (47.0881, 52.5084) -> (33.6537, 52.5084)
  line L1390 (47.0881, 52.5084) -> (33.6537, 52.5084)
  line L1391 (47.0881, 52.5084) -> (33.6537, 52.5084)
  line L1392 (47.0881, 52.5084) -> (33.6537, 52.5084)
  line L1393 (33.6537, 48.5084) -> (47.0881, 48.5084)
  line L1394 (33.6537, 48.5084) -> (47.0881, 48.5084)
  line L1395 (33.6537, 48.5084) -> (47.0881, 48.5084)
  arc A1570 (13.6537, 52.5084) -> (13.6537, 48.5084) centre (13.6537, 50.5084) ccw
  arc A1571 (13.6537, 52.5084) -> (13.6537, 48.5084) centre (13.6537, 50.5084) ccw
  arc A1572 (13.6537, 52.5084) -> (13.6537, 48.5084) centre (13.6537, 50.5084) ccw
  arc A1573 (13.6537, 52.5084) -> (13.6537, 48.5084) centre (13.6537, 50.5084) ccw
  arc A1574 (13.6537, 52.5084) -> (13.6537, 48.5084) centre (13.6537, 50.5084) ccw
  arc A1575 (13.6537, 52.5084) -> (13.6537, 48.5084) centre (13.6537, 50.5084) ccw
  arc A1576 (7.0881, 48.5084) -> (7.0881, 52.5084) centre (7.0881, 50.5084) ccw
  arc A1577 (7.0881, 48.5084) -> (7.0881, 52.5084) centre (7.0881, 50.5084) ccw
  arc A1578 (7.0881, 48.5084) -> (7.0881, 52.5084) centre (7.0881, 50.5084) ccw
  arc A1579 (7.0881, 48.5084) -> (7.0881, 52.5084) centre (7.0881, 50.5084) ccw
  arc A1580 (17.5876, 55.4654) -> (17.5876, 59.4654) centre (17.5876, 57.4654) ccw
  arc A1581 (17.5876, 55.4654) -> (17.5876, 59.4654) centre (17.5876, 57.4654) ccw
  arc A1582 (17.5876, 55.4654) -> (17.5876, 59.4654) centre (17.5876, 57.4654) ccw
  arc A1583 (17.5876, 55.4654) -> (17.5876, 59.4654) centre (17.5876, 57.4654) ccw
  arc A1584 (17.5876, 55.4654) -> (17.5876, 59.4654) centre (17.5876, 57.4654) ccw
  arc A1585 (17.5876, 55.4654) -> (17.5876, 59.4654) centre (17.5876, 57.4654) ccw
  arc A1586 (24.1532, 59.4654) -> (24.1532, 55.4654) centre (24.1532, 57.4654) ccw
  arc A1587 (24.1532, 59.4654) -> (24.1532, 55.4654) centre (24.1532, 57.4654) ccw
  arc A1588 (24.1532, 59.4654) -> (24.1532, 55.4654) centre (24.1532, 57.4654) ccw
  arc A1589 (24.1532, 59.4654) -> (24.1532, 55.4654) centre (24.1532, 57.4654) ccw
  arc A1590 (24.1532, 59.4654) -> (24.1532, 55.4654) centre (24.1532, 57.4654) ccw
  arc A1591 (24.1532, 59.4654) -> (24.1532, 55.4654) centre (24.1532, 57.4654) ccw
  arc A1592 (24.1532, 59.4654) -> (24.1532, 55.4654) centre (24.1532, 57.4654) ccw
  arc A1593 (24.1532, 59.4654) -> (24.1532, 55.4654) centre (24.1532, 57.4654) ccw
  arc A1594 (24.1532, 59.4654) -> (24.1532, 55.4654) centre (24.1532, 57.4654) ccw
  arc A1595 (4.1532, 59.4654) -> (4.1532, 55.4654) centre (4.1532, 57.4654) ccw
  arc A1596 (4.1532, 59.4654) -> (4.1532, 55.4654) centre (4.1532, 57.4654) ccw
  arc A1597 (4.1532, 59.4654) -> (4.1532, 55.4654) centre (4.1532, 57.4654) ccw
  arc A1598 (4.1532, 59.4654) -> (4.1532, 55.4654) centre (4.1532, 57.4654) ccw
  arc A1599 (4.1532, 59.4654) -> (4.1532, 55.4654) centre (4.1532, 57.4654) ccw
  arc A1600 (4.1532, 59.4654) -> (4.1532, 55.4654) centre (4.1532, 57.4654) ccw
  arc A1601 (4.1532, 59.4654) -> (4.1532, 55.4654) centre (4.1532, 57.4654) ccw
  arc A1602 (4.1532, 59.4654) -> (4.1532, 55.4654) centre (4.1532, 57.4654) ccw
  arc A1603 (4.1532, 59.4654) -> (4.1532, 55.4654) centre (4.1532, 57.4654) ccw
  arc A1604 (-2.4124, 55.4654) -> (-2.4124, 59.4654) centre (-2.4124, 57.4654) ccw
  arc A1605 (-2.4124, 55.4654) -> (-2.4124, 59.4654) centre (-2.4124, 57.4654) ccw
  arc A1606 (-2.4124, 55.4654) -> (-2.4124, 59.4654) centre (-2.4124, 57.4654) ccw
  arc A1607 (-2.4124, 55.4654) -> (-2.4124, 59.4654) centre (-2.4124, 57.4654) ccw
  arc A1608 (-32.9119, 48.5084) -> (-32.9119, 52.5084) centre (-32.9119, 50.5084) ccw
  arc A1609 (-32.9119, 48.5084) -> (-32.9119, 52.5084) centre (-32.9119, 50.5084) ccw
  arc A1610 (-32.9119, 48.5084) -> (-32.9119, 52.5084) centre (-32.9119, 50.5084) ccw
  arc A1611 (-32.9119, 48.5084) -> (-32.9119, 52.5084) centre (-32.9119, 50.5084) ccw
  arc A1612 (-32.9119, 48.5084) -> (-32.9119, 52.5084) centre (-32.9119, 50.5084) ccw
  arc A1613 (-32.9119, 48.5084) -> (-32.9119, 52.5084) centre (-32.9119, 50.5084) ccw
  line L1396 (27.0881, 52.5084) -> (13.6537, 52.5084)
  line L1397 (13.6537, 48.5084) -> (27.0881, 48.5084)
  line L1398 (27.0881, 52.5084) -> (13.6537, 52.5084)
  line L1399 (13.6537, 48.5084) -> (27.0881, 48.5084)
  line L1400 (13.6537, 48.5084) -> (27.0881, 48.5084)
  line L1401 (27.0881, 52.5084) -> (13.6537, 52.5084)
  line L1402 (27.0881, 52.5084) -> (13.6537, 52.5084)
  line L1403 (27.0881, 52.5084) -> (13.6537, 52.5084)
  line L1404 (13.6537, 48.5084) -> (27.0881, 48.5084)
  line L1405 (13.6537, 48.5084) -> (27.0881, 48.5084)
  line L1406 (13.6537, 48.5084) -> (27.0881, 48.5084)
  line L1407 (27.0881, 52.5084) -> (13.6537, 52.5084)
  line L1408 (4.1532, 55.4654) -> (17.5876, 55.4654)
  line L1409 (4.1532, 55.4654) -> (17.5876, 55.4654)
  line L1410 (4.1532, 55.4654) -> (17.5876, 55.4654)
  line L1411 (4.1532, 55.4654) -> (17.5876, 55.4654)
  line L1412 (4.1532, 55.4654) -> (17.5876, 55.4654)
  line L1413 (4.1532, 55.4654) -> (17.5876, 55.4654)
  line L1414 (17.5876, 59.4654) -> (4.1532, 59.4654)
  line L1415 (17.5876, 59.4654) -> (4.1532, 59.4654)
  line L1416 (17.5876, 59.4654) -> (4.1532, 59.4654)
  line L1417 (17.5876, 59.4654) -> (4.1532, 59.4654)
  line L1418 (17.5876, 59.4654) -> (4.1532, 59.4654)
  line L1419 (17.5876, 59.4654) -> (4.1532, 59.4654)
  arc A1614 (7.0881, 48.5084) -> (7.0881, 52.5084) centre (7.0881, 50.5084) ccw
  arc A1615 (7.0881, 48.5084) -> (7.0881, 52.5084) centre (7.0881, 50.5084) ccw
  line L1420 (-6.3463, 48.5084) -> (7.0881, 48.5084)
  line L1421 (7.0881, 52.5084) -> (-6.3463, 52.5084)
  line L1422 (7.0881, 52.5084) -> (-6.3463, 52.5084)
  line L1423 (-6.3463, 48.5084) -> (7.0881, 48.5084)
  line L1424 (-6.3463, 48.5084) -> (7.0881, 48.5084)
  line L1425 (7.0881, 52.5084) -> (-6.3463, 52.5084)
  line L1426 (7.0881, 52.5084) -> (-6.3463, 52.5084)
  line L1427 (7.0881, 52.5084) -> (-6.3463, 52.5084)
  line L1428 (-6.3463, 48.5084) -> (7.0881, 48.5084)
  line L1429 (-6.3463, 48.5084) -> (7.0881, 48.5084)
  line L1430 (-6.3463, 48.5084) -> (7.0881, 48.5084)
  line L1431 (7.0881, 52.5084) -> (-6.3463, 52.5084)
  arc A1616 (-6.3463, 52.5084) -> (-6.3463, 48.5084) centre (-6.3463, 50.5084) ccw
  arc A1617 (-6.3463, 52.5084) -> (-6.3463, 48.5084) centre (-6.3463, 50.5084) ccw
  arc A1618 (-6.3463, 52.5084) -> (-6.3463, 48.5084) centre (-6.3463, 50.5084) ccw
  arc A1619 (-6.3463, 52.5084) -> (-6.3463, 48.5084) centre (-6.3463, 50.5084) ccw
  arc A1620 (-6.3463, 52.5084) -> (-6.3463, 48.5084) centre (-6.3463, 50.5084) ccw
  arc A1621 (-6.3463, 52.5084) -> (-6.3463, 48.5084) centre (-6.3463, 50.5084) ccw
  arc A1622 (-12.9119, 48.5084) -> (-12.9119, 52.5084) centre (-12.9119, 50.5084) ccw
  arc A1623 (-12.9119, 48.5084) -> (-12.9119, 52.5084) centre (-12.9119, 50.5084) ccw
  arc A1624 (-12.9119, 48.5084) -> (-12.9119, 52.5084) centre (-12.9119, 50.5084) ccw
  arc A1625 (-12.9119, 48.5084) -> (-12.9119, 52.5084) centre (-12.9119, 50.5084) ccw
  arc A1626 (-12.9119, 48.5084) -> (-12.9119, 52.5084) centre (-12.9119, 50.5084) ccw
  line L1432 (-2.4124, 59.4654) -> (-15.8468, 59.4654)
  line L1433 (-15.8468, 55.4654) -> (-2.4124, 55.4654)
  line L1434 (-2.4124, 59.4654) -> (-15.8468, 59.4654)
  line L1435 (-15.8468, 55.4654) -> (-2.4124, 55.4654)
  line L1436 (-2.4124, 59.4654) -> (-15.8468, 59.4654)
  line L1437 (-15.8468, 55.4654) -> (-2.4124, 55.4654)
  line L1438 (-2.4124, 59.4654) -> (-15.8468, 59.4654)
  line L1439 (-15.8468, 55.4654) -> (-2.4124, 55.4654)
  line L1440 (-2.4124, 59.4654) -> (-15.8468, 59.4654)
  line L1441 (-15.8468, 55.4654) -> (-2.4124, 55.4654)
  line L1442 (-15.8468, 55.4654) -> (-2.4124, 55.4654)
  line L1443 (-2.4124, 59.4654) -> (-15.8468, 59.4654)
  arc A1627 (-2.4124, 55.4654) -> (-2.4124, 59.4654) centre (-2.4124, 57.4654) ccw
  arc A1628 (-2.4124, 55.4654) -> (-2.4124, 59.4654) centre (-2.4124, 57.4654) ccw
  arc A1629 (-15.8468, 59.4654) -> (-15.8468, 55.4654) centre (-15.8468, 57.4654) ccw
  arc A1630 (-15.8468, 59.4654) -> (-15.8468, 55.4654) centre (-15.8468, 57.4654) ccw
  arc A1631 (-15.8468, 59.4654) -> (-15.8468, 55.4654) centre (-15.8468, 57.4654) ccw
  arc A1632 (-15.8468, 59.4654) -> (-15.8468, 55.4654) centre (-15.8468, 57.4654) ccw
  arc A1633 (-15.8468, 59.4654) -> (-15.8468, 55.4654) centre (-15.8468, 57.4654) ccw
  arc A1634 (-22.4124, 55.4654) -> (-22.4124, 59.4654) centre (-22.4124, 57.4654) ccw
  arc A1635 (-22.4124, 55.4654) -> (-22.4124, 59.4654) centre (-22.4124, 57.4654) ccw
  arc A1636 (-15.8468, 59.4654) -> (-15.8468, 55.4654) centre (-15.8468, 57.4654) ccw
  arc A1637 (-15.8468, 59.4654) -> (-15.8468, 55.4654) centre (-15.8468, 57.4654) ccw
  arc A1638 (-22.4124, 55.4654) -> (-22.4124, 59.4654) centre (-22.4124, 57.4654) ccw
  arc A1639 (-15.8468, 59.4654) -> (-15.8468, 55.4654) centre (-15.8468, 57.4654) ccw
  arc A1640 (-15.8468, 59.4654) -> (-15.8468, 55.4654) centre (-15.8468, 57.4654) ccw
  arc A1641 (-22.4124, 55.4654) -> (-22.4124, 59.4654) centre (-22.4124, 57.4654) ccw
  arc A1642 (-22.4124, 55.4654) -> (-22.4124, 59.4654) centre (-22.4124, 57.4654) ccw
  arc A1643 (-22.4124, 55.4654) -> (-22.4124, 59.4654) centre (-22.4124, 57.4654) ccw
  arc A1644 (-26.3463, 52.5084) -> (-26.3463, 48.5084) centre (-26.3463, 50.5084) ccw
  arc A1645 (-26.3463, 52.5084) -> (-26.3463, 48.5084) centre (-26.3463, 50.5084) ccw
  arc A1646 (-26.3463, 52.5084) -> (-26.3463, 48.5084) centre (-26.3463, 50.5084) ccw
  arc A1647 (-26.3463, 52.5084) -> (-26.3463, 48.5084) centre (-26.3463, 50.5084) ccw
  arc A1648 (-26.3463, 52.5084) -> (-26.3463, 48.5084) centre (-26.3463, 50.5084) ccw
  arc A1649 (-26.3463, 52.5084) -> (-26.3463, 48.5084) centre (-26.3463, 50.5084) ccw
  line L1444 (-35.8468, 55.4654) -> (-22.4124, 55.4654)
  line L1445 (-35.8468, 55.4654) -> (-22.4124, 55.4654)
  line L1446 (-35.8468, 55.4654) -> (-22.4124, 55.4654)
  line L1447 (-35.8468, 55.4654) -> (-22.4124, 55.4654)
  line L1448 (-35.8468, 55.4654) -> (-22.4124, 55.4654)
  line L1449 (-35.8468, 55.4654) -> (-22.4124, 55.4654)
  line L1450 (-22.4124, 59.4654) -> (-35.8468, 59.4654)
  line L1451 (-22.4124, 59.4654) -> (-35.8468, 59.4654)
  line L1452 (-22.4124, 59.4654) -> (-35.8468, 59.4654)
  line L1453 (-22.4124, 59.4654) -> (-35.8468, 59.4654)
  line L1454 (-22.4124, 59.4654) -> (-35.8468, 59.4654)
  line L1455 (-22.4124, 59.4654) -> (-35.8468, 59.4654)
  line L1456 (-26.3463, 48.5084) -> (-12.9119, 48.5084)
  line L1457 (-12.9119, 52.5084) -> (-26.3463, 52.5084)
  line L1458 (-12.9119, 52.5084) -> (-26.3463, 52.5084)
  line L1459 (-26.3463, 48.5084) -> (-12.9119, 48.5084)
  line L1460 (-12.9119, 52.5084) -> (-26.3463, 52.5084)
  line L1461 (-12.9119, 52.5084) -> (-26.3463, 52.5084)